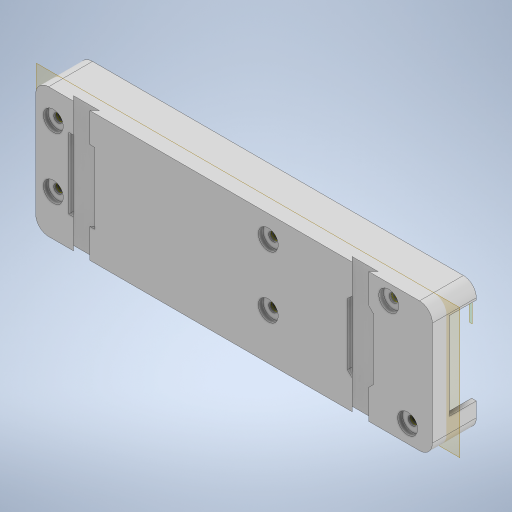
# Autodesk Inventor part: osmobuddy_bottom
Saved by Autodesk Inventor 2024.3 (Build 283343000, 343)
## iProperties
Created: 2024-08-31
Part Number: osmobuddy_bottom
Material: Generic
Document SubType Name: Modeling
Designer: atrus
Density: 1 g/cm^3
Appearance: Default
Author: atrus
Autodesk Inventor part; units mm, degrees
ref_plane "YZ Plane" through (0, 0, 0) normal (1, 0, 0) x (0, 1, 0)
ref_plane "XZ Plane" through (0, 0, 0) normal (0, 1, 0) x (-1, 0, 0)
ref_plane "Work Plane1" through (0, 0, 0) normal (0, 0, 1) x (1, 0, 0)
ref_plane "Work Plane2" through (-64.2976, -17.57, -1.1916) normal (0, 0, 1) x (1, 0, 0)
sketch "Sketch1" plane through (0, 0, 0) normal (0, 0, 1) x (1, 0, 0)
  line L0 (78.5, 25) -> (-78.5, 25) construction
  arc A0 (-78.5, 25) -> (-81.5, 22) centre (-78.5, 22) ccw construction
  line L1 (-81.5, 22) -> (-81.5, -22) construction
  arc A1 (-81.5, -22) -> (-78.5, -25) centre (-78.5, -22) ccw construction
  line L2 (-78.5, -25) -> (78.5, -25) construction
  arc A2 (78.5, -25) -> (81.5, -22) centre (78.5, -22) ccw construction
  line L3 (81.5, -22) -> (81.5, 22) construction
  arc A3 (81.5, 22) -> (78.5, 25) centre (78.5, 22) ccw construction
  line L4 (-78.5, 25.5) -> (78.5, 25.5)
  arc A4 (82, 22) -> (78.5, 25.5) centre (78.5, 22) ccw
  line L5 (82, 22) -> (82, -22)
  arc A5 (78.5, -25.5) -> (82, -22) centre (78.5, -22) ccw
  line L6 (78.5, -25.5) -> (-78.5, -25.5)
  arc A6 (-82, -22) -> (-78.5, -25.5) centre (-78.5, -22) ccw
  line L7 (-82, -22) -> (-82, 22)
  arc A7 (-78.5, 25.5) -> (-82, 22) centre (-78.5, 22) ccw
  line L8 (78.5, 27.45) -> (-78.5, 27.45)
  arc A8 (-78.5, 27.45) -> (-83.95, 22) centre (-78.5, 22) ccw
  line L9 (-83.95, 22) -> (-83.95, -22)
  arc A9 (-83.95, -22) -> (-78.5, -27.45) centre (-78.5, -22) ccw
  line L10 (-78.5, -27.45) -> (78.5, -27.45)
  arc A10 (78.5, -27.45) -> (83.95, -22) centre (78.5, -22) ccw
  line L11 (83.95, -22) -> (83.95, 22)
  arc A11 (83.95, 22) -> (78.5, 27.45) centre (78.5, 22) ccw
  point P0 (0, 0)
  dimension "d0" = 0.5
  dimension "d1" = 1.95
  constraints: 16 end point, 16 point on circle, 8 centre point, 14 other
  measures "d0" distance between parallel lines of L4 L0
  measures "d1" distance between parallel lines of L8 L4
extrude "Extrusion2" add sketch "Sketch1" against normal up to surface (1.1916 mm away)
sketch "Sketch3" plane through (0, 0, 0) normal (0, 0, 1) x (1, 0, 0)
  arc A0 (-78.5, 27.45) -> (-83.95, 22) centre (-78.5, 22) ccw projected
  line L0 (-83.95, 22) -> (-83.95, -22) projected
  arc A1 (-83.95, -22) -> (-78.5, -27.45) centre (-78.5, -22) ccw projected
  line L1 (-78.5, -27.45) -> (78.5, -27.45) projected
  arc A2 (78.5, -27.45) -> (83.95, -22) centre (78.5, -22) ccw projected
  line L2 (83.95, -22) -> (83.95, 22) projected
  arc A3 (83.95, 22) -> (78.5, 27.45) centre (78.5, 22) ccw projected
  line L3 (78.5, 27.45) -> (-78.5, 27.45) projected
  line L4 (-82, -22) -> (-82, 22) projected
  arc A4 (-78.5, 25.5) -> (-82, 22) centre (-78.5, 22) ccw projected
  line L5 (-78.5, 25.5) -> (78.5, 25.5) projected
  arc A5 (82, 22) -> (78.5, 25.5) centre (78.5, 22) ccw projected
  line L6 (82, 22) -> (82, -22) projected
  arc A6 (78.5, -25.5) -> (82, -22) centre (78.5, -22) ccw projected
  line L7 (78.5, -25.5) -> (-78.5, -25.5) projected
  arc A7 (-82, -22) -> (-78.5, -25.5) centre (-78.5, -22) ccw projected
  point P0 (0, 0)
extrude "Extrusion3" add sketch "Sketch3" along normal blind 3
sketch "Sketch4" plane through (0, 0, 3) normal (0, 0, 1) x (1, 0, 0)
  line L0 (78.5, 27.45) -> (-78.5, 27.45) projected
  arc A0 (-78.5, 27.45) -> (-83.95, 22) centre (-78.5, 22) ccw projected
  line L1 (-83.95, 22) -> (-83.95, -22) projected
  arc A1 (-83.95, -22) -> (-78.5, -27.45) centre (-78.5, -22) ccw projected
  line L2 (-78.5, -27.45) -> (78.5, -27.45) projected
  arc A2 (78.5, -27.45) -> (83.95, -22) centre (78.5, -22) ccw projected
  line L3 (83.95, -22) -> (83.95, 22) projected
  arc A3 (83.95, 22) -> (78.5, 27.45) centre (78.5, 22) ccw projected
  point P0 (0, 0)
extrude "Extrusion4" add sketch "Sketch4" along normal blind 3
ref_plane "Work Plane3" through (70.3002, 20.9998, -12.598) normal (0, 0, -1) x (1, 0, 0)
sketch "Sketch5" plane through (78.5, -27.45, -1.1916) normal (0, 0, -1) x (-1, 0.0000001, 0)
  arc A0 (160.5, 49.45) -> (157, 52.95) centre (157, 49.45) ccw projected
  line L0 (160.5, 49.45) -> (160.5, 5.45) projected
  arc A1 (157, 1.95) -> (160.5, 5.45) centre (157, 5.45) ccw projected
  line L1 (157, 1.95) -> (0, 1.95) projected
  arc A2 (-3.5, 5.45) -> (0, 1.95) centre (0, 5.45) ccw projected
  line L2 (-3.5, 5.45) -> (-3.5, 49.45) projected
  arc A3 (0, 52.95) -> (-3.5, 49.45) centre (0, 49.45) ccw projected
  line L3 (0, 52.95) -> (157, 52.95) projected
  line L4 (162.45, 5.45) -> (162.45, 49.45) projected
  arc A4 (162.45, 49.45) -> (157, 54.9) centre (157, 49.45) ccw projected
  line L5 (157, 54.9) -> (0, 54.9) projected
  arc A5 (0, 54.9) -> (-5.45, 49.45) centre (0, 49.45) ccw projected
  line L6 (-5.45, 49.45) -> (-5.45, 5.45) projected
  arc A6 (-5.45, 5.45) -> (0, 0) centre (0, 5.45) ccw projected
  line L7 (0, 0) -> (157, 0) projected
  arc A7 (157, 0) -> (162.45, 5.45) centre (157, 5.45) ccw projected
  point P0 (78.5, 27.45)
extrude "Extrusion5" add sketch "Sketch5" along normal up to surface (11.4064 mm away)
sketch "Sketch6" plane through (-78.5, -27.45, 6) normal (-0.0000001, -1, 0) x (1, -0.0000001, 0)
  line L0 (146.741, -6.0075) -> (146.741, -13.4075) construction
  line L1 (134.521, -6.0075) -> (134.521, -13.4075) construction
  line L2 (130.741, -6.0075) -> (130.741, -13.4075) construction
  line L3 (118.491, -6.3075) -> (118.491, -12.3075) construction
  line L4 (116.741, -12.3075) -> (116.741, -6.7075) construction
  line L5 (104.491, -6.3075) -> (104.491, -12.3075) construction
  line L6 (102.741, -12.3075) -> (102.741, -6.7075) construction
  line L7 (90.491, -6.3075) -> (90.491, -12.3075) construction
  line L8 (87.17, -12.9495) -> (87.17, -5.1495) construction
  line L9 (78.76, -12.9495) -> (78.76, -5.1495) construction
  line L10 (68.76, -12.9495) -> (68.76, -5.1495) construction
  line L11 (58.76, -12.9495) -> (58.76, -5.1495) construction
  line L12 (77.17, -12.9495) -> (77.17, -5.1495) construction
  line L13 (67.17, -12.9495) -> (67.17, -5.1495) construction
  line L14 (53.98, -12.9495) -> (53.98, -5.1495) construction
  line L15 (43.98, -12.9495) -> (43.98, -5.1495) construction
  line L16 (35.57, -4.0495) -> (35.57, -10.2495) construction
  line L17 (33.98, -12.9495) -> (33.98, -5.1495) construction
  line L18 (23.98, -12.9495) -> (23.98, -5.1495) construction
  line L19 (13.741, -12.3075) -> (13.741, -6.7075) construction
  line L20 (45.57, -12.9495) -> (45.57, -5.1495) construction
  line L21 (35.57, -12.9495) -> (35.57, -5.1495) construction
  line L22 (23.98, -4.0495) -> (23.98, -10.2495) construction
  line L23 (25.57, -12.9495) -> (25.57, -5.1495) construction
  line L24 (15.57, -12.9495) -> (15.57, -5.1495) construction
  line L25 (1.491, -6.3075) -> (1.491, -12.3075) construction
  line L26 (142.953, -6.0075) -> (146.741, -6.0075) construction
  line L27 (0, -18.598) -> (157, -18.598) projected
  line L28 (146.941, -18.598) -> (134.321, -18.598)
  line L29 (134.321, -18.598) -> (134.321, -7.7575)
  line L30 (134.321, -7.7575) -> (146.941, -7.7575)
  line L31 (146.941, -7.7575) -> (146.941, -18.598)
  line L32 (0, -18.598) -> (157, -18.598) projected
  line L33 (130.941, -7.7575) -> (118.291, -7.7575)
  line L34 (118.291, -7.7575) -> (118.291, -18.598)
  line L35 (118.291, -18.598) -> (130.941, -18.598)
  line L36 (130.941, -18.598) -> (130.941, -7.7575)
  line L37 (116.941, -7.7575) -> (104.291, -7.7575)
  line L38 (104.291, -7.7575) -> (104.291, -18.598)
  line L39 (104.291, -18.598) -> (116.941, -18.598)
  line L40 (116.941, -18.598) -> (116.941, -7.7575)
  line L41 (102.941, -7.7575) -> (90.291, -7.7575)
  line L42 (90.291, -7.7575) -> (90.291, -18.598)
  line L43 (90.291, -18.598) -> (102.941, -18.598)
  line L44 (102.941, -18.598) -> (102.941, -7.7575)
  line L45 (87.37, -7.7575) -> (78.5, -7.7575)
  line L46 (78.5, -7.7575) -> (78.5, -18.598)
  line L47 (78.5, -18.598) -> (87.37, -18.598)
  line L48 (87.37, -18.598) -> (87.37, -7.7575)
  line L49 (77.37, -7.7575) -> (68.56, -7.7575)
  line L50 (68.56, -7.7575) -> (68.56, -18.598)
  line L51 (68.56, -18.598) -> (77.37, -18.598)
  line L52 (77.37, -18.598) -> (77.37, -7.7575)
  line L53 (67.37, -7.7575) -> (58.56, -7.7575)
  line L54 (58.56, -7.7575) -> (58.56, -18.598)
  line L55 (58.56, -18.598) -> (67.37, -18.598)
  line L56 (67.37, -18.598) -> (67.37, -7.7575)
  line L57 (54.18, -7.7575) -> (45.37, -7.7575)
  line L58 (45.37, -7.7575) -> (45.37, -18.598)
  line L59 (45.37, -18.598) -> (54.18, -18.598)
  line L60 (54.18, -18.598) -> (54.18, -7.7575)
  line L61 (44.18, -7.7575) -> (35.37, -7.7575)
  line L62 (35.37, -7.7575) -> (35.37, -18.598)
  line L63 (35.37, -18.598) -> (44.18, -18.598)
  line L64 (44.18, -18.598) -> (44.18, -7.7575)
  line L65 (34.18, -7.7575) -> (25.37, -7.7575)
  line L66 (25.37, -7.7575) -> (25.37, -18.598)
  line L67 (25.37, -18.598) -> (34.18, -18.598)
  line L68 (34.18, -18.598) -> (34.18, -7.7575)
  line L69 (24.18, -7.7575) -> (15.37, -7.7575)
  line L70 (15.37, -7.7575) -> (15.37, -18.598)
  line L71 (15.37, -18.598) -> (24.18, -18.598)
  line L72 (24.18, -18.598) -> (24.18, -7.7575)
  line L73 (13.941, -7.7575) -> (1.291, -7.7575)
  line L74 (1.291, -7.7575) -> (1.291, -18.598)
  line L75 (1.291, -18.598) -> (13.941, -18.598)
  line L76 (13.941, -18.598) -> (13.941, -7.7575)
  line L77 (146.741, -6.0075) -> (146.741, -13.4075) projected
  line L78 (145.929, -8.7575) -> (145.3897, -8.7575) projected
  point P0 (78.5, -6)
  point P1 (144.847, -6.0075)
  point P2 (23.98, -9.0495)
  point P3 (13.941, -18.598)
  point P4 (102.941, -18.598)
  point P5 (116.941, -18.598)
  point P6 (130.941, -18.598)
  point P7 (145.6594, -8.7575)
  dimension "d12" = 0.2
  dimension "d13" = 0.2
  dimension "d15" = 0.2
  dimension "d16" = 0.2
  dimension "d17" = 0.2
  dimension "d18" = 0.2
  dimension "d19" = 0.2
  dimension "d20" = 0.2
  dimension "d21" = 0.2
  dimension "d22" = 0.2
  dimension "d23" = 0.2
  dimension "d24" = 0.2
  dimension "d25" = 0.2
  dimension "d26" = 0.2
  dimension "d27" = 0.2
  dimension "d28" = 0.2
  dimension "d29" = 0.2
  dimension "d30" = 0.2
  dimension "d31" = 0.2
  dimension "d32" = 0.2
  dimension "d33" = 0.2
  dimension "d34" = 0.2
  dimension "d35" = 0.2
  dimension "d81" = 1
  constraints: 96 end point, 24 parallel, 12 horizontal, 12 perpendicular, 10 point on line, 3 midpoint, 1 collinear, 14 other
  measures "d12" distance between parallel lines of L31 L0
  measures "d13" distance between parallel lines of L29 L1
  measures "d15" distance between parallel lines of L2 L36
  measures "d16" distance between parallel lines of L34 L3
  measures "d17" distance between parallel lines of L40 L4
  measures "d18" distance between parallel lines of L5 L38
  measures "d19" distance between parallel lines of L44 L6
  measures "d20" distance between parallel lines of L7 L42
  measures "d21" distance between parallel lines of L48 L8
  measures "d22" distance between parallel lines of L52 L12
  measures "d23" distance between parallel lines of L50 L10
  measures "d24" distance between parallel lines of L13 L56
  measures "d25" distance between parallel lines of L54 L11
  measures "d26" distance between parallel lines of L14 L60
  measures "d27" distance between parallel lines of L15 L64
  measures "d28" distance between parallel lines of L17 L68
  measures "d29" distance from line of point (23.98, -9.049) L72
  measures "d30" distance between parallel lines of L19 L76
  measures "d31" distance between parallel lines of L20 L58
  measures "d32" distance between parallel lines of L21 L62
  measures "d33" distance between parallel lines of L23 L66
  measures "d34" distance between parallel lines of L24 L70
  measures "d35" distance between parallel lines of L25 L74
  measures "d81" distance from line of point (145.659, -8.757) L30
extrude "Extrusion6" cut sketch "Sketch6" against normal blind 10
sketch "Sketch7" plane through (83.95, -22, 6) normal (1, 0, 0) x (0, 0, -1)
  line L0 (18.3948, 42.9998) -> (7.3948, 42.9998) construction
  line L1 (7.3948, 42.9998) -> (7.3948, 33.9998) construction
  line L2 (7.3948, 33.9998) -> (18.3948, 33.9998) construction
  line L3 (18.3948, 33.9998) -> (18.3948, 42.9998) construction
  circle A0 centre (13.8948, 38.4998) radius 3.25 construction
  line L4 (15.2148, 31.6672) -> (15.2148, 21.8328) construction
  line L5 (7.9548, 21.8328) -> (7.9548, 31.6672) construction
  line L6 (15.2148, 17.9172) -> (15.2148, 8.0828) construction
  line L7 (7.9048, 17.9824) -> (7.9048, 8.0176) construction
  line L8 (7.9548, 17.9172) -> (15.2148, 17.9172) construction
  line L9 (14.0148, 21.8595) -> (8.9248, 21.8595) construction
  line L10 (7.9548, 31.6672) -> (15.2148, 31.6672) construction
  line L11 (14.0148, 8.1095) -> (8.9248, 8.1095) construction
  line L12 (18.598, 0) -> (18.598, 44) construction
  line L13 (7.1948, 43.1998) -> (18.598, 43.1998)
  line L14 (18.598, 43.1998) -> (18.598, 33.7998)
  line L15 (7.1948, 33.7998) -> (7.1948, 43.1998)
  line L16 (12.4848, 6.425) -> (15.2148, 6.425) projected
  line L17 (18.598, 33.7998) -> (18.598, 6.225)
  line L18 (7.1948, 33.7998) -> (7.1948, 6.225)
  line L19 (7.1948, 6.225) -> (18.598, 6.225)
  point P0 (13.8498, 6.425)
  dimension "d45" = 0.2
  dimension "d47" = 0.2
  dimension "d82" = 0.2
  constraints: 12 end point, 2 perpendicular, 2 point on line, 1 horizontal, 1 midpoint, 1 parallel, 1 vertical
  measures "d45" distance between parallel lines of L13 L0
  measures "d47" distance between parallel lines of L1 L15
  measures "d82" vertical distance of L17.end point (13.85, 6.425)
extrude "Extrusion7" cut sketch "Sketch7" against normal blind 10
sketch "Sketch8" plane through (-83.95, -22, 6) normal (-1, 0.0000002, 0) x (0, 0, 1)
  arc A0 (-9.3748, 29.054) -> (-10.6548, 27.774) centre (-9.3748, 27.774) ccw construction
  line L0 (-10.6548, 21.394) -> (-10.6548, 27.774) construction
  arc A1 (-10.6548, 21.394) -> (-9.3748, 20.114) centre (-9.3748, 21.394) ccw construction
  line L1 (-9.3748, 20.114) -> (-8.7748, 20.114) projected
  arc A2 (-8.7748, 20.114) -> (-7.4948, 21.394) centre (-8.7748, 21.394) ccw construction
  line L2 (-7.4948, 21.394) -> (-7.4948, 24.329) construction
  line L3 (-7.4948, 24.329) -> (-7.6948, 24.329) projected
  line L4 (-7.6948, 24.329) -> (-7.6948, 21.394) construction
  arc A3 (-8.7748, 20.314) -> (-7.6948, 21.394) centre (-8.7748, 21.394) ccw construction
  line L5 (-8.7748, 20.314) -> (-9.3748, 20.314) projected
  arc A4 (-10.4548, 21.394) -> (-9.3748, 20.314) centre (-9.3748, 21.394) ccw construction
  line L6 (-10.4548, 21.394) -> (-10.4548, 27.774) construction
  arc A5 (-9.3748, 28.854) -> (-10.4548, 27.774) centre (-9.3748, 27.774) ccw construction
  line L7 (-9.3748, 28.854) -> (-8.7748, 28.854) construction
  arc A6 (-7.6948, 27.774) -> (-8.7748, 28.854) centre (-8.7748, 27.774) ccw construction
  line L8 (-7.6948, 27.774) -> (-7.6948, 24.339) construction
  line L9 (-7.6948, 24.339) -> (-7.4948, 24.339) projected
  line L10 (-7.4948, 24.339) -> (-7.4948, 27.774) construction
  arc A7 (-7.4948, 27.774) -> (-8.7748, 29.054) centre (-8.7748, 27.774) ccw construction
  line L11 (-8.7748, 29.054) -> (-9.3748, 29.054) construction
  line L12 (-7.8948, 21.394) -> (-7.8948, 24.529)
  line L13 (-7.8948, 24.529) -> (-7.2948, 24.529) construction
  line L14 (-7.2948, 24.529) -> (-7.2948, 21.394)
  arc A8 (-8.7748, 19.914) -> (-7.2948, 21.394) centre (-8.7748, 21.394) ccw
  line L15 (-8.7748, 19.914) -> (-9.3748, 19.914)
  line L16 (-9.3748, 29.254) -> (-8.7748, 29.254)
  arc A9 (-7.2948, 27.774) -> (-8.7748, 29.254) centre (-8.7748, 27.774) ccw
  line L17 (-7.2948, 27.774) -> (-7.2948, 24.139)
  line L18 (-7.2948, 24.139) -> (-7.8948, 24.139) construction
  line L19 (-7.8948, 24.139) -> (-7.8948, 27.774)
  line L20 (-18.598, 44) -> (-18.598, 0) projected
  line L21 (-9.3748, 29.254) -> (-18.598, 29.254)
  line L22 (-9.3748, 19.914) -> (-18.598, 19.914)
  line L23 (-18.598, 19.914) -> (-18.598, 29.254)
  point P0 (-6, 22)
  point P1 (-9.0748, 29.254)
  dimension "d50" = 0.2
  constraints: 22 end point, 4 point on circle, 3 perpendicular, 2 centre point, 2 point on line, 1 midpoint, 8 other
  measures "d50" distance from line of point (-9.075, 29.254) L11
extrude "Extrusion8" cut sketch "Sketch8" against normal blind 10
sketch "Sketch10" plane through (0, 0, 6) normal (0, 0, 1) x (1, 0, 0)
  circle A0 centre (73.5, -20) radius 1.7 projected
  circle A1 centre (65.5, 21) radius 1.7 projected
  circle A2 centre (14.5, 18) radius 1.7 projected
  circle A3 centre (14.5, -8) radius 1.7 projected
  circle A4 centre (-76.5, -10) radius 1.7 projected
  circle A5 centre (-76.5, 16) radius 1.7 projected
  point P0 (0, 0)
hole "Hole1" at (65.5, 21, 6) at (73.5, -20, 6) at (14.5, 18, 6) at (14.5, -8, 6) at (-76.5, 16, 6) at (-76.5, -10, 6) direction (0, 0, -1) diameter 3.6 end through all counterbore diameter 8.4 counterbore depth 2 clearance for "Hex Head Machine Screw" size "M3" standard "Ansi Metric M Profile"
sketch "Sketch11" plane through (0, 0, 3) normal (0, 0, -1) x (-1, 0, 0)
  circle A0 centre (-14.5, 18) radius 4.2 projected
  circle A1 centre (-14.5, 18) radius 1.7 projected
  circle A2 centre (-14.5, -8) radius 4.2 projected
  circle A3 centre (-14.5, -8) radius 1.7 projected
  circle A4 centre (76.5, -10) radius 4.2 projected
  circle A5 centre (76.5, -10) radius 1.7 projected
  circle A6 centre (76.5, 16) radius 4.2 projected
  circle A7 centre (76.5, 16) radius 1.7 projected
  circle A8 centre (-73.5, -20) radius 4.2 projected
  circle A9 centre (-73.5, -20) radius 1.7 projected
  circle A10 centre (-65.5, 21) radius 4.2 projected
  circle A11 centre (-65.5, 21) radius 1.7 projected
  point P0 (0, 0)
extrude "Extrusion9" add sketch "Sketch11" along normal blind 3
sketch "Sketch12" plane through (0, 0, 3) normal (0, 0, -1) x (-1, 0, 0)
  circle A0 centre (-67.5, -2) radius 1.7 projected
  circle A1 centre (-67.5, -2) radius 1.5
  point P0 (0, 0)
  dimension "d62" = 0.2
  constraints: 1 centre point, 1 coincident
  measures "d62" radial gap between concentric circles of A0 A1
ref_plane "Work Plane4" through (-81.5, -25, -1.4202) normal (0, 0, -1) x (0, 1, 0)
extrude "Extrusion10" add sketch "Sketch12" along normal up to surface (4.4202 mm away) contours A1
sketch "Sketch13" plane through (0, 0, 3) normal (0, 0, -1) x (-1, 0, 0)
  circle A0 centre (-58.01, 18.476) radius 1.524 construction
  circle A1 centre (-27.53, 18.476) radius 1.524 construction
  circle A2 centre (-27.53, -9.464) radius 1.524 construction
  circle A3 centre (-58.01, -9.464) radius 1.524 construction
  circle A4 centre (-27.53, 18.476) radius 1.324
  circle A5 centre (-27.53, -9.464) radius 1.324
  circle A6 centre (-58.01, -9.464) radius 1.324
  circle A7 centre (-58.01, 18.476) radius 1.324
  point P0 (0, 0)
  dimension "d65" = 0.2
  constraints: 4 centre point, 4 coincident, 3 equal radius
  measures "d65" radial gap between concentric circles of A1 A4
extrude "Extrusion11" add sketch "Sketch13" along normal blind 14.732
chamfer "Chamfer1" distance 2 angle 45 11 edges at (28.854, 18.476, 3) (28.854, -9.464, 3) (59.334, -9.464, 3) (59.334, 18.476, 3) (69.7, 21, 3) (69, -2, 3) (18.7, 18, 3) (18.7, -8, 3) (-72.3, 16, 3) (-72.3, -10, 3) (77.7, -20, 3)
sketch "Sketch14" plane through (-78.5, 27.45, 6) normal (0.0000001, 1, 0) x (1, -0.0000001, 0)
  line L0 (135.5, 0) -> (137.5, 2)
  line L1 (137.5, 2) -> (126.5, 2)
  line L2 (126.5, 2) -> (128.5, 0)
  line L3 (128.5, 0) -> (135.5, 0)
  line L4 (157, 0) -> (0, 0) construction
  line L5 (17.5, 0) -> (19.5, 2)
  line L6 (19.5, 2) -> (8.5, 2)
  line L7 (8.5, 2) -> (10.5, 0)
  line L8 (10.5, 0) -> (17.5, 0)
  line L9 (157, 18.598) -> (157, 0) projected
  point P0 (132, 0)
  point P1 (132, 2)
  point P2 (14, 2)
  point P3 (39, 0)
  point P4 (14, 0)
  dimension "d72" = 7
  dimension "d77" = 135
  dimension "d84" = 2
  dimension "d87" = 118
  dimension "d92" = 25
  constraints: 16 end point, 3 point on line, 2 midpoint, 1 horizontal, 1 parallel, 1 perpendicular, 11 other
  measures "d72" distance of L2.end L0.start
  measures "d77" angle of L1 L0
  measures "d84" distance of point (132, 2) point (132, 0)
  measures "d87" distance of L0.start L5.start
  measures "d92" distance from line of L9 point (132, 2)
extrude "Extrusion12" cut sketch "Sketch14" against normal through all
chamfer "Chamfer2" distance 1 angle 45 5 edges at (-83.95, -1.6525, -1.7282) (-83.95, -2.086, -7.6864) (-83.95, 2.584, -1.2948) (-83.95, 6.8205, -1.7282) (-83.95, 7.254, -7.6864)
sketch "Sketch15" plane through (0, 0, 6) normal (0, 0, 1) x (1, 0, 0)
  line L0 (-68, -27.45) -> (-68, 27.45) projected
  line L1 (-61, 27.45) -> (-61, -27.45) projected
  line L2 (-59, 27.45) -> (-59, -27.45) projected
  line L3 (-70, 27.45) -> (-70, -27.45) projected
  line L4 (50, -27.45) -> (50, 27.45) projected
  line L5 (57, 27.45) -> (57, -27.45) projected
  line L6 (59, 27.45) -> (59, -27.45) projected
  line L7 (48, 27.45) -> (48, -27.45) projected
  line L8 (-70, 15) -> (-68, 15)
  line L9 (-61, 15) -> (-59, 15)
  line L10 (-70, -15) -> (-68, -15)
  line L11 (-61, -15) -> (-59, -15)
  line L12 (48, 15) -> (50, 15)
  line L13 (57, 15) -> (59, 15)
  line L14 (48, -15) -> (50, -15)
  line L15 (57, -15) -> (59, -15)
  line L16 (-68, 0) -> (59, 0) construction
  point P0 (0, 0)
  point P1 (-60, 15)
  point P2 (-60, -15)
  point P3 (49, 15)
  point P4 (-69, 15)
  dimension "d93" = 15
  dimension "d94" = 15
  dimension "d95" = 15
  dimension "d96" = 15
  constraints: 24 point on line, 18 end point, 6 midpoint, 3 perpendicular, 1 horizontal
  measures "d93" distance from line of L16 point (-60, 15)
  measures "d94" distance from line of L16 point (-60, -15)
  measures "d95" distance from line of point (49, 15) L16
  measures "d96" distance from line of L16 point (-69, 15)
extrude "Extrusion13" cut sketch "Sketch15" against normal blind 2
chamfer "Chamfer4" distance 1.99 angle 45 4 edges at (59, -15, 5) (48, -15, 5) (59, 15, 5) (48, 15, 5)
body "Solid2"
